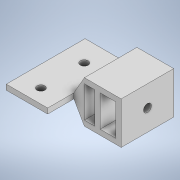
# Autodesk Inventor part: VbearingBracket
Saved by Autodesk Inventor 2020 (Build 240168000, 168)
## iProperties
Created: 2020-01-12
Part Number: VbearingBracket
Material: Generic
Document SubType Name: Modeling
Designer: tdmp4
Density: 1 g/cm^3
Appearance: Default
Author: tdmp4
Autodesk Inventor part; units mm, degrees
ref_plane "YZ Plane" through (0, 0, 0) normal (1, 0, 0) x (0, 1, 0)
ref_plane "XZ Plane" through (0, 0, 0) normal (0, 1, 0) x (-1, 0, 0)
ref_plane "XY Plane" through (0, 0, 0) normal (0, 0, 1) x (1, 0, 0)
sketch "Sketch1" plane through (0, 0, 0) normal (0, 1, 0) x (-1, 0, 0)
  line L0 (0, -27.8975) -> (20, -27.8975)
  line L1 (20, -27.8975) -> (20, -53.2975)
  line L2 (20, -53.2975) -> (0, -53.2975)
  line L3 (0, -53.2975) -> (0, -27.8975)
  point P0 (0, 0)
  dimension "d0" = 20
  dimension "d1" = 25.4
  constraints: 8 end point, 2 parallel, 1 horizontal, 1 perpendicular
  measures "d0" distance of L1.end L2.end
  measures "d1" distance of L2.end L0.start
extrude "Extrusion1" add sketch "Sketch1" along normal blind 2.54
sketch "Sketch2" plane through (0, 0, -27.8975) normal (1, 0, 0) x (0, 0, -1)
  line L0 (0, 0) -> (25.4, 0) projected
  line L1 (0, 2.54) -> (25.4, 2.54)
  line L2 (25.4, 2.54) -> (25.4, 0)
  line L3 (25.4, 0) -> (0, 0)
  line L4 (0, 0) -> (0, 2.54)
  point P0 (-27.8975, 0)
  constraints: 8 end point, 2 parallel, 1 horizontal, 1 perpendicular
extrude "Extrusion2" add sketch "Sketch2" along normal blind 5.08
sketch "Sketch4" plane through (-20, 0, -27.8975) normal (0, 0, 1) x (1, 0, 0)
  line L0 (25.08, 2.54) -> (25.08, 0) construction
  line L1 (25.08, 2.54) -> (20, 2.54) construction
  line L2 (0, 0) -> (25.08, 0) projected
  line L3 (25.08, 0) -> (20, 0)
  line L4 (0, 2.54) -> (25.08, 2.54) projected
  line L5 (25.08, 2.54) -> (25.08, 11.43)
  line L6 (25.08, 0) -> (25.08, -8.89)
  line L7 (20, 2.54) -> (25.08, 11.43)
  line L8 (20, 0) -> (25.08, -8.89)
  line L9 (25.08, 11.43) -> (40.32, 11.43)
  line L10 (40.32, 11.43) -> (40.32, 8.898)
  line L11 (40.32, 8.898) -> (25.08, 8.898)
  line L12 (25.08, 8.898) -> (25.08, 11.43)
  line L13 (25.08, -8.89) -> (40.32, -8.89)
  line L14 (40.32, -8.89) -> (40.32, -6.3453)
  line L15 (40.32, -6.3453) -> (25.08, -6.3453)
  line L16 (25.08, -6.3453) -> (25.08, -8.89)
  line L17 (33.4394, 8.898) -> (30.8868, 8.898)
  line L18 (30.8868, -6.3453) -> (33.4394, -6.3453)
  line L19 (40.32, 11.43) -> (42.8586, 11.43)
  line L20 (42.8586, 11.43) -> (42.8586, -8.89)
  line L21 (42.8586, -8.89) -> (40.32, -8.89)
  line L22 (40.32, -8.89) -> (40.32, 11.43)
  line L23 (32.7, -6.3453) -> (30.1586, -6.3453)
  line L24 (30.1586, -6.3453) -> (30.1586, 8.898)
  line L25 (30.1586, 8.898) -> (32.7, 8.898)
  line L26 (32.7, 8.898) -> (32.7, -6.3453)
  dimension "d6" = 8.89
  dimension "d7" = 2.54
  dimension "d9" = 8.89
  dimension "d10" = 15.24
  dimension "d16" = 15.24
  constraints: 48 end point, 9 parallel, 7 horizontal, 5 perpendicular, 5 point on line, 1 vertical
  measures "d6" distance of L0.start L5.end
  measures "d7" distance of L0.start L0.end
  measures "d9" distance of L0.end L6.end
  measures "d10" distance of L5.end L9.end
  measures "d16" distance of L14.end L15.end
extrude "Extrusion3" add sketch "Sketch4" against normal blind 25.4 contours L2 L6 L8 | L6 L15 L14 L13 | L14 L22 L10 L19 L20 L21 | L24 L11 L26 L15 | L11 L5 L9 L10 | L5 L4 L7
sketch "Sketch6" plane through (22.8586, -8.89, -27.8975) normal (1, 0, 0) x (0, 0, -1)
  line L0 (25.4, 11.43) -> (25.4, 20.32) projected
  line L1 (0, 8.89) -> (0, 0) projected
  line L2 (25.4, 20.32) -> (0, 20.32)
  line L3 (0, 20.32) -> (0, 0)
  line L4 (0, 0) -> (25.4, 0)
  line L5 (25.4, 0) -> (25.4, 20.32)
  line L6 (0, 20.32) -> (0, 11.43) projected
  line L7 (25.4, 0) -> (0, 20.32)
  line L8 (0, 0) -> (25.4, 20.32)
  circle A0 centre (12.7, 10.16) radius 1.905
  point P0 (-27.8975, 8.89)
  dimension "d17" = 3.81
  constraints: 12 end point, 2 parallel, 1 centre point, 1 horizontal, 1 midpoint, 1 perpendicular
  measures "d17" diameter of A0
extrude "Extrusion5" cut sketch "Sketch6" against normal blind 14.2875 contours A0 L7 L8 | L8 L7 A0 | A0 L8 L7 | L7 L8 A0
sketch "Sketch7" plane through (0, 2.54, 0) normal (0, 1, 0) x (1, 0, 0)
  line L0 (-20, 27.8975) -> (0, 27.8975) projected
  line L1 (0, 27.8975) -> (0, 53.2975) projected
  line L2 (-20, 27.8975) -> (0, 27.8975)
  line L3 (0, 27.8975) -> (0, 42.8975)
  line L4 (0, 42.8975) -> (-20, 42.8975)
  line L5 (-20, 42.8975) -> (-20, 27.8975)
  circle A0 centre (-10, 42.8975) radius 1.905
  point P0 (0, 0)
  dimension "d20" = 15
  dimension "d21" = 3.81
  constraints: 8 end point, 2 parallel, 1 centre point, 1 horizontal, 1 midpoint, 1 perpendicular, 1 point on line
  measures "d20" distance of L4.end L0.start
  measures "d21" diameter of A0
extrude "Extrusion6" cut sketch "Sketch7" against normal blind 28.575 contours A0 L4 | L4 A0
sketch "Sketch8" plane through (-20, 0, -27.8975) normal (0, 0, 1) x (1, 0, 0)
  line L0 (0, 0) -> (20, 0) projected
  line L1 (0, 2.54) -> (20, 2.54) projected
  line L2 (0, 0) -> (20, 0)
  line L3 (20, 0) -> (20, 2.54)
  line L4 (20, 2.54) -> (0, 2.54)
  line L5 (0, 2.54) -> (0, 0)
  constraints: 8 end point, 2 parallel, 1 horizontal, 1 perpendicular
extrude "Extrusion7" add sketch "Sketch8" along normal blind 12.7
sketch "Sketch9" plane through (0, 2.54, 0) normal (0, 1, 0) x (1, 0, 0)
  circle A0 centre (-10, 21.9147) radius 1.905
  point P0 (0, 0)
  dimension "d26" = 3.81
  constraints: 1 centre point
  measures "d26" diameter of A0
extrude "Extrusion8" cut sketch "Sketch9" against normal blind 76.2
body "Solid1"
